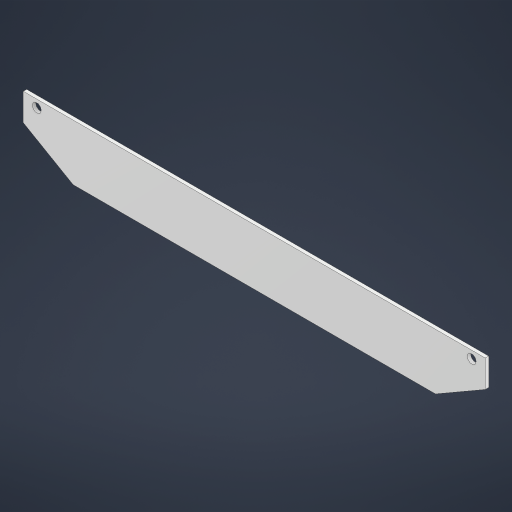
# Autodesk Inventor part: wedge
Saved by Autodesk Inventor 2024 (Build 280153000, 153)
## iProperties
Created: 2023-11-21
Part Number: wedge
Material: Acetal Resin, White
Document SubType Name: Sheet Metal
Designer: avere
Density: 1.425 g/cm^3
Appearance: Smooth - White
Flat Pattern Width: 2.61471 cm
Flat Pattern Length: 21.59 cm
Flat Pattern Area: 56.4515 cm^2
Sheet Metal Rule: Default_mm
Sheet Metal Width: 1.029 in
Sheet Metal Length: 8.500 in
Sheet Metal Area: 8.750 in^2
Author: avere
Autodesk Inventor part; units mm, degrees
ref_plane "YZ Plane" through (0, 0, 0) normal (1, 0, 0) x (0, 1, 0)
ref_plane "XZ Plane" through (0, 0, 0) normal (0, 1, 0) x (-1, 0, 0)
ref_plane "XY Plane" through (0, 0, 0) normal (0, 0, 1) x (1, 0, 0)
sketch "Block1" plane through (0, 0, 0) normal (0, 0, 1) x (1, 0, 0)
  line L0 (-105.9874, 13.2259) -> (-105.9874, 0.5259)
  line L1 (109.9126, 13.2259) -> (-105.9874, 13.2259)
  line L2 (109.9126, 0.5259) -> (109.9126, 13.2259)
  line L3 (86.6216, -12.9211) -> (-82.6964, -12.9211)
  line L4 (-105.9874, 0.5259) -> (-82.6964, -12.9211)
  line L5 (109.9126, 0.5259) -> (86.6216, -12.9211)
  circle A0 centre (-99.6374, 9.7141) radius 2.0955
  circle A1 centre (103.5626, 9.7141) radius 2.0955
  point P0 (3.9065, 11.282)
  dimension "d30" = 4.191
  dimension "d31" = 4.191
  measures "d30" diameter of A0
  measures "d31" diameter of A1
sketch "Sketch1" plane through (0, 0, 0) normal (0, 0, 1) x (1, 0, 0)
  line L0 (-6.35, -6.35) -> (-6.35, -19.05)
  line L1 (209.55, -6.35) -> (-6.35, -6.35)
  line L2 (209.55, -19.05) -> (209.55, -6.35)
  line L3 (186.259, -32.4971) -> (16.941, -32.4971)
  line L4 (-6.35, -19.05) -> (16.941, -32.4971)
  line L5 (209.55, -19.05) -> (186.259, -32.4971)
  circle A0 centre (0, -9.8618) radius 2.0955
  circle A1 centre (203.2, -9.8618) radius 2.0955
  point P0 (0, 0)
extrude "Extrusion1" add sketch "Sketch1" along normal blind 1.5875
feature "Bend Part1" [suppressed]
equation "\"BendRadius\" = Thickness"
equation "\"BendReliefWidth\" = Thickness"
equation "\"BendReliefDepth\" = 0.5 * Thickness"
equation "\"CornerReliefSize\" = 4 * Thickness"
equation "\"MinimumRemnant\" = 2 * Thickness"
equation "\"TransitionRadius\" = BendRadius"
equation "\"JacobiRadiusSize\" = BendRadius"
equation "\"GapSize\" = Thickness"
equation "\"Thickness\" = 1.5875"
body "Solid1"
